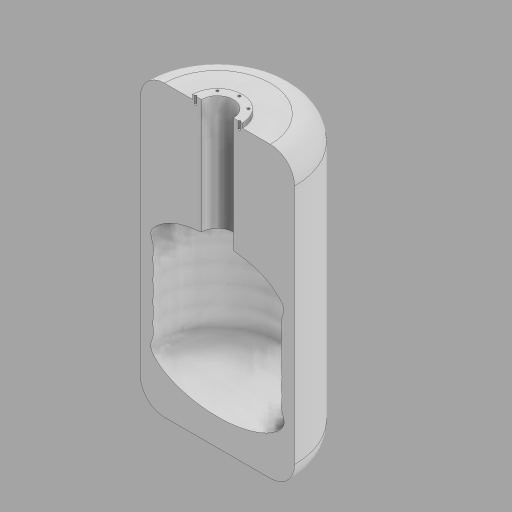
# Autodesk Inventor part: TransportDewar
Saved by Autodesk Inventor 2024 (Build 280153020, 153B)
## iProperties
Created: 2023-10-25
Part Number: TransportDewar
Material: Generic
Document SubType Name: Modeling
Designer: schanen
Density: 1 g/cm^3
Appearance: Default
Author: schanen
Autodesk Inventor part; units mm, degrees
ref_plane "YZ Plane" through (0, 0, 0) normal (1, 0, 0) x (0, 1, 0)
ref_plane "XZ Plane" through (0, 0, 0) normal (0, 1, 0) x (-1, 0, 0)
ref_plane "XY Plane" through (0, 0, 0) normal (0, 0, 1) x (1, 0, 0)
sketch "InnerShape" plane through (0, 0, 0) normal (0, 0, 1) x (1, 0, 0)
  spline S0 degree 4 poles (25.5438, 42.0281) (88.3985, 41.1205) (175.7883, 56.4516) (240.2524, 85.3572) (289.1446, 125.5476) (307.0428, 154.2136) (298.3402, 181.4897) (286.4701, 206.6436) (294.5788, 232.4697) (293.8632, 257.9202) (288.0995, 283.3382) (294.0239, 308.6783) (294.0576, 334.1754) (288.0277, 359.5276) (294.0484, 384.8821) (294.0529, 410.3743) (288.018, 435.7273) (294.0857, 461.094) (293.9522, 486.6266) (288.2436, 512.1618) (293.3771, 538.0681) (309.1971, 564.4637) (288.3219, 593.5581) (240.7199, 632.9003) (183.1395, 665.8542) (80.5578, 674.6739) (25.5438, 677.0281) knots 0 0 0 0 0 0.143858 0.187431 0.224823 0.259091 0.291676 0.323874 0.356024 0.388045 0.420047 0.452068 0.484088 0.516091 0.548112 0.580132 0.612135 0.644156 0.676226 0.708422 0.741006 0.775272 0.812434 0.855963 1 1 1 1 1
  point P0 (254.729, 359.5281)
  point P1 (142.9438, 54.7281)
  point P2 (219.4438, 80.1281)
  point P3 (263.0438, 105.5281)
  point P4 (290.4438, 130.9281)
  point P5 (302.0438, 156.3281)
  point P6 (297.4438, 181.7281)
  point P7 (290.4438, 207.1281)
  point P8 (292.8438, 232.5281)
  point P9 (292.8438, 257.9281)
  point P10 (290.4438, 283.3281)
  point P11 (292.8438, 308.7281)
  point P12 (292.8438, 334.1281)
  point P13 (290.4438, 359.5281)
  point P14 (292.8438, 384.9281)
  point P15 (292.8438, 410.3281)
  point P16 (290.4438, 435.7281)
  point P17 (292.8438, 461.1281)
  point P18 (292.8438, 486.5281)
  point P19 (290.4438, 511.9281)
  point P20 (295.1438, 537.3281)
  point P21 (302.0438, 562.7281)
  point P22 (290.4438, 588.1281)
  point P23 (263.0438, 613.5281)
  point P24 (222.6438, 638.9281)
  point P25 (142.9438, 664.3281)
sketch "Sketch2" plane through (0, 0, 0) normal (0, 0, 1) x (1, 0, 0)
  line L0 (66.5, 630.0055) -> (66.5, 1106)
  line L1 (66.5, 1106) -> (103.5, 1106)
  line L2 (103.5, 1106) -> (103.5, 1088)
  line L3 (103.5, 1088) -> (220, 1088)
  line L4 (320, 988) -> (320, -12)
  line L5 (220, -112) -> (0, -112)
  line L6 (0, -112) -> (0, 0)
  arc A0 (320, 988) -> (220, 1088) centre (220, 988) ccw
  arc A1 (220, -112) -> (320, -12) centre (220, -12) ccw
  spline S0 degree 4 poles (0, 0) (62.8547, -0.9075) (150.2445, 14.4235) (214.7086, 43.3291) (263.6008, 83.5195) (281.499, 112.1856) (272.7964, 139.4616) (260.9263, 164.6155) (269.035, 190.4417) (268.3194, 215.8922) (262.5557, 241.3102) (268.4801, 266.6503) (268.5138, 292.1474) (262.4839, 317.4996) (268.5046, 342.854) (268.5091, 368.3463) (262.4742, 393.6993) (268.5419, 419.0659) (268.4084, 444.5985) (262.6998, 470.1338) (267.8333, 496.04) (283.6534, 522.4356) (262.7781, 551.5301) (215.1761, 590.8722) (157.5957, 623.8262) (55.014, 632.6458) (0, 635) knots 0 0 0 0 0 0.143858 0.187431 0.224823 0.259091 0.291676 0.323874 0.356024 0.388045 0.420047 0.452068 0.484088 0.516091 0.548112 0.580132 0.612135 0.644156 0.676226 0.708422 0.741006 0.775272 0.812434 0.855963 1 1 1 1 1
  point P0 (320, 1088)
  point P1 (320, -112)
  point P2 (0, 0)
  dimension "d9" = 1106
  dimension "d10" = 66.5
  dimension "d11" = 103.5
  dimension "d12" = 320
  dimension "d13" = 18
  dimension "d14" = 1200
  dimension "d15" = 100
  dimension "d16" = 100
  constraints: 14 end point, 4 perpendicular, 4 point on circle, 4 point on line, 4 tangent, 2 centre point, 2 vertical, 1 horizontal, 3 other
  measures "d10" distance of the line from the sketch origin of L0
  measures "d11" distance of the line from the sketch origin of L2
  measures "d12" distance of the line from the sketch origin of L4
  measures "d13" distance of L1.end L2.end
  measures "d14" distance of point (320, 1088) point (320, -112)
  measures "d15" radius of A0
  measures "d16" radius of A1
revolve "Revolution1" add sketch "Sketch2" angle 360 about axis through (0, -112, 0) along (0, 1, 0)
sketch "Sketch3" plane through (0, 1106, 0) normal (0, 1, 0) x (1, 0, 0)
  point P0 (0, 0)
  point P1 (0, 91)
  dimension "d18" = 91
  measures "d18" distance of point (0, 0) point (0, 91)
hole "Hole1" at (0, 1106, -91) direction (0, -1, 0) diameter 10.106 depth 30 tip angle 118 thread size "M12x1.75" class "6H" standard "ISO Metric profile"
pattern_circular "Circular Pattern1" count 8 over 360 about axis through (0, 868.0028, 0) along (0, 1, 0) of "Hole1"
sketch "Sketch5" plane through (0, 1106, 0) normal (0, 1, 0) x (1, 0, 0)
  circle A0 centre (0, 0) radius 320 projected
  line L0 (-320, 0) -> (320, 0)
  line L1 (320, 0) -> (320, -320)
  line L2 (320, -320) -> (-320, -320)
  line L3 (-320, -320) -> (-320, 0)
  point P0 (0, -320)
  constraints: 8 end point, 2 parallel, 1 horizontal, 1 perpendicular, 2 other
extrude "Extrusion2" cut sketch "Sketch5" against normal through all contours A0 L0 | A0 L2 L3 picked at (-65.063, -184.508)
body "Solid1"
